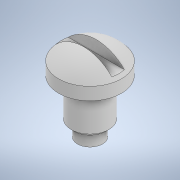
# Autodesk Inventor part: parafuso_de_trava
Saved by Autodesk Inventor 2022 (Build 260153000, 153)
## iProperties
Created: 2022-03-09
Part Number: parafuso_de_trava
Material: Generic
Document SubType Name: Modeling
Designer: Korch
Density: 1 g/cm^3
Appearance: Default
Author: Korch
Autodesk Inventor part; units mm, degrees
ref_plane "YZ Plane" through (0, 0, 0) normal (1, 0, 0) x (0, 1, 0)
ref_plane "XZ Plane" through (0, 0, 0) normal (0, 1, 0) x (-1, 0, 0)
ref_plane "XY Plane" through (0, 0, 0) normal (0, 0, 1) x (1, 0, 0)
sketch "Sketch2" plane through (0, 0, 0) normal (0, 0, 1) x (1, 0, 0)
  arc A0 (5, 3.75) -> (-5, 3.75) centre (0, 0) ccw
  line L0 (0, 3.75) -> (5, 3.75)
  line L1 (0, 3.75) -> (-5, 3.75)
  line L2 (5, 3.75) -> (5, 1.75)
  line L3 (-5, 1.75) -> (-5, 3.75)
  line L4 (-5, 1.75) -> (-2, 1.75)
  line L5 (2.5391, 1.25) -> (2.5391, 1.75)
  line L6 (-2.2609, 1.25) -> (-2.2609, 1.75)
  line L7 (0, -6.75) -> (2, -6.75)
  line L8 (0, -6.75) -> (-2, -6.75)
  line L9 (-2, -6.75) -> (-2, -4.75)
  line L10 (2, -6.75) -> (2, -4.75)
  line L11 (-3, -4.25) -> (-3, 1.25)
  line L12 (-3, 1.25) -> (-2.2609, 1.25)
  line L13 (2.5391, 1.25) -> (3, 1.25)
  line L14 (3, 1.25) -> (3, -4.25)
  line L15 (-2, -4.75) -> (-2.5, -4.75)
  line L16 (-2.5, -4.75) -> (-2.9403, -4.3097)
  line L17 (-2.5, -4.75) -> (-1.8773, -4.75) construction
  line L18 (-2.9403, -4.3097) -> (-3, -4.25)
  line L19 (2, -4.75) -> (2.5, -4.75)
  line L20 (2.5, -4.75) -> (3, -4.25)
  line L21 (5, 1.75) -> (2.5391, 1.75)
  line L22 (-2.2609, 1.75) -> (-5, 1.75)
  line L23 (0, 6.25) -> (0, -6.75)
  dimension "d10" = 0.5
  dimension "d15" = 2
  dimension "d16" = 2
  dimension "d20" = 0.5
  dimension "d23" = 135
  dimension "d24" = 0.5
  dimension "d25" = 135
  constraints: 48 end point, 9 perpendicular, 4 horizontal, 4 point on line, 3 point on circle, 3 vertical, 1 centre point, 1 coincident, 1 equal length
  measures "d10" distance of L5.start L5.end
  measures "d15" distance of L7.start L7.end
  measures "d16" distance of L7.start L8.end
  measures "d20" distance of L9.end L15.end
  measures "d23" angle of L17 L16
  measures "d24" distance of L10.end L19.end
  measures "d25" angle of L20 L19
revolve "Revolution1" add sketch "Sketch2" angle 360 about axis through (0, 6.25, 0) along (0, -1, 0) contours L23 L1 A0 | L23 L8 L9 L15 L16 L18 L11 L12 L6 L4 L3 L1
ref_plane "Work Plane1" through (0, 6.25, 0) normal (0, -1, 0) x (1, 0, 0)
sketch "Sketch3" plane through (0, 6.25, 0) normal (0, -1, 0) x (1, 0, 0)
  circle A0 centre (0, 0) radius 5
  line L0 (0, 1) -> (-4.899, 1)
  circle A1 centre (0, 0) radius 5 projected
  line L1 (-4.899, -1) -> (0, -1)
  line L2 (0, -1) -> (5.6598, -1)
  line L3 (5.6598, -1) -> (5.6598, 1)
  line L4 (5.6598, 1) -> (0, 1)
  line L5 (-4.899, 1) -> (-6.6915, 1)
  line L6 (-6.6915, 1) -> (-6.6915, -1)
  line L7 (-6.6915, -1) -> (-4.899, -1)
  point P0 (4.899, 1)
  point P1 (4.899, -1)
  constraints: 16 end point, 2 perpendicular, 2 point on line, 1 coincident, 1 collinear, 1 horizontal, 5 other
extrude "Extrusion1" cut sketch "Sketch3" along normal blind 2 contours L0 L4 A0 L2 L1
body "Solid1"
